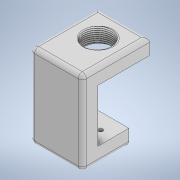
# Autodesk Inventor part: Clamp_Main_Body
Saved by Autodesk Inventor 2021 (Build 250183000, 183)
## iProperties
Created: 2021-04-05
Part Number: Clamp_Main_Body
Material: Generic
Document SubType Name: Modeling
Designer: Ariel Wolle
Density: 1 g/cm^3
Appearance: Default
Author: Ariel Wolle
Autodesk Inventor part; units mm, degrees
ref_plane "YZ Plane" through (0, 0, 0) normal (1, 0, 0) x (0, 1, 0)
ref_plane "XZ Plane" through (0, 0, 0) normal (0, 1, 0) x (-1, 0, 0)
ref_plane "XY Plane" through (0, 0, 0) normal (0, 0, 1) x (1, 0, 0)
sketch "Sketch1" plane through (0, 0, 0) normal (0, 0, 1) x (1, 0, 0)
  line L0 (130, -15) -> (80, -15)
  line L1 (80, -15) -> (80, 27.7)
  line L2 (80, 27.7) -> (130, 27.7)
  line L3 (130, 27.7) -> (130, -15)
  point P0 (0, 0)
  dimension "d0" = 42.7
  dimension "d1" = 15
  dimension "d2" = 80
  dimension "d3" = 50
  constraints: 8 end point, 2 parallel, 1 horizontal, 1 perpendicular
  measures "d0" distance of L2.end L0.start
  measures "d1" distance from line of point (0, 0) L0
  measures "d2" distance from line of point (0, 0) L1
  measures "d3" distance of L0.start L0.end
extrude "Extrusion1" add sketch "Sketch1" along normal blind 15
sketch "Sketch2" plane through (0, 0, 0) normal (0, 0, -1) x (-1, 0, 0)
  line L0 (-80, -15) -> (-130, -15) projected
  line L1 (-80, 27.7) -> (-80, -15) projected
  line L2 (-130, -15) -> (-80, -15)
  line L3 (-80, -15) -> (-80, 0)
  line L4 (-80, 0) -> (-130, 0)
  line L5 (-130, 0) -> (-130, -15)
  point P0 (0, 0)
  constraints: 8 end point, 2 parallel, 1 horizontal, 1 perpendicular, 1 point on line
extrude "Extrusion2" add sketch "Sketch2" along normal blind 30
sketch "Sketch3" plane through (80, -15, 15) normal (0, -1, 0) x (1, 0, 0)
  circle A0 centre (12, -29.7778) radius 2
  circle A1 centre (38, -29.7778) radius 2.1598
  line L0 (0, -45) -> (0, 0) projected
  line L1 (50, -45) -> (50, 0) projected
  point P0 (-80, -15)
  dimension "d8" = 4
  dimension "d9" = 12
  dimension "d10" = 12
  constraints: 2 centre point
  measures "d8" diameter of A0
  measures "d9" distance from line of L0 A0.centre
  measures "d10" distance from line of L1 A1.centre
extrude "Extrusion3" cut sketch "Sketch3" against normal blind 30
chamfer "Chamfer1" distance 2 angle 45 2 edges at (90, -15, -14.7778) (115.8402, -15, -14.7778)
fillet "Fillet1" radius 4 1 edges at (105, -15, 15)
sketch "Sketch4" plane through (80, 27.7, 0) normal (0, 1, 0) x (1, 0, 0)
  line L0 (50, -11) -> (50, -15) projected
  line L1 (0, 0) -> (0, 30) projected
  line L2 (50, -15) -> (0, -15)
  line L3 (0, -15) -> (0, 0)
  line L4 (0, 0) -> (50, 0)
  line L5 (50, 0) -> (50, -15)
  point P0 (-80, 0)
  constraints: 8 end point, 2 parallel, 1 horizontal, 1 perpendicular
extrude "Extrusion4" add sketch "Sketch4" along normal blind 23.1
sketch "Sketch5" plane through (80, 50.8, 0) normal (0, 1, 0) x (1, 0, 0)
  line L0 (0, -15) -> (0, -11) projected
  line L1 (50, 0) -> (50, 30) projected
  line L2 (0, -15) -> (50, -15)
  line L3 (50, -15) -> (50, 0)
  line L4 (50, 0) -> (0, 0)
  line L5 (0, 0) -> (0, -15)
  point P0 (-80, 0)
  point P1 (0, -11)
  constraints: 8 end point, 2 parallel, 1 horizontal, 1 perpendicular
extrude "Extrusion5" add sketch "Sketch5" along normal blind 15
sketch "Sketch6" plane through (0, 0, 0) normal (0, 0, -1) x (-1, 0, 0)
  line L0 (-130, 65.8) -> (-80, 65.8) projected
  line L1 (-130, 0) -> (-130, 65.8) projected
  line L2 (-80, 65.8) -> (-130, 65.8)
  line L3 (-130, 65.8) -> (-130, 50.8)
  line L4 (-130, 50.8) -> (-80, 50.8)
  line L5 (-80, 50.8) -> (-80, 65.8)
  point P0 (0, 0)
  dimension "d21" = 15
  constraints: 8 end point, 2 parallel, 1 horizontal, 1 perpendicular, 1 point on line
  measures "d21" distance between parallel lines of L4 L0
extrude "Extrusion6" add sketch "Sketch6" along normal blind 50
sketch "Sketch7" plane through (80, 65.8, 0) normal (0, 1, 0) x (1, 0, 0)
  line L0 (0, 50) -> (50, 50) projected
  line L1 (0, -15) -> (0, 50) projected
  circle A0 centre (25, 25) radius 13.5
  point P0 (-80, 0)
  dimension "d32" = 25
  dimension "d33" = 25
  dimension "d34" = 27
  constraints: 1 centre point, 1 coincident
  measures "d32" distance from line of L0 point (25, 25)
  measures "d33" distance from line of L1 point (25, 25)
  measures "d34" diameter of A0
fillet "Fillet2" radius 4 11 edges at (105, 65.8, 15) (80, 65.8, -17.5) (130, 65.8, -17.5) (105, 65.8, -50) (80, -13.8284, 13.8284) (80, -15, -9.5) (80, 27.4, 15) (130, -13.8284, 13.8284) (130, -15, -9.5) (130, 27.4, 15) (105, -15, -30)
extrude "Extrusion7" cut sketch "Sketch7" against normal up to surface (15 mm away)
ref_plane "Work Plane2" through (0, 0, -25) normal (0, 0, -1) x (-1, 0, 0)
sketch "Sketch8" plane through (0, 0, -25) normal (0, 0, -1) x (-1, 0, 0)
  line L0 (-80, 50.8) -> (-130, 50.8) construction
  line L1 (-89.4629, 50.8) -> (-89.4629, 66.2032) construction
  line L2 (-80, 50.8) -> (-130, 50.8) construction
  line L3 (-130, 0) -> (-130, 50.8) construction
  line L4 (-130, 0) -> (-80, 0) construction
  line L5 (-80, 0) -> (-80, 50.8) construction
  line L6 (-80, 50.8) -> (-80, 61.8) construction
  arc A0 (-126, 65.8) -> (-130, 61.8) centre (-126, 61.8) ccw construction
  line L7 (-126, 65.8) -> (-118.5, 65.8) construction
  line L8 (-118.5, 65.8) -> (-118.5, 50.8) construction
  line L9 (-118.5, 50.8) -> (-130, 50.8) construction
  line L10 (-130, 50.8) -> (-130, 61.8) construction
  arc A1 (-80, 61.8) -> (-84, 65.8) centre (-84, 61.8) ccw construction
  line L11 (-80, 61.8) -> (-80, 50.8) construction
  line L12 (-80, 50.8) -> (-91.5, 50.8) construction
  line L13 (-91.5, 50.8) -> (-91.5, 65.8) construction
  line L14 (-91.5, 65.8) -> (-84, 65.8) construction
  arc A2 (-130, -11) -> (-126, -15) centre (-126, -11) ccw construction
  line L15 (-130, -11) -> (-130, 0) construction
  line L16 (-130, 0) -> (-80, 0) construction
  line L17 (-80, 0) -> (-80, -11) construction
  arc A3 (-84, -15) -> (-80, -11) centre (-84, -11) ccw construction
  line L18 (-84, -15) -> (-126, -15) construction
  arc A4 (-126, 65.8) -> (-130, 61.8) centre (-126, 61.8) ccw construction
  line L19 (-126, 65.8) -> (-118.5, 65.8) construction
  line L20 (-118.5, 50.8) -> (-130, 50.8) construction
  line L21 (-130, 50.8) -> (-130, 61.8) construction
  arc A5 (-80, 61.8) -> (-84, 65.8) centre (-84, 61.8) ccw construction
  line L22 (-80, 61.8) -> (-80, 50.8) construction
  line L23 (-80, 50.8) -> (-91.5, 50.8) construction
  line L24 (-91.5, 65.8) -> (-84, 65.8) construction
  arc A6 (-130, -11) -> (-126, -15) centre (-126, -11) ccw construction
  line L25 (-130, -11) -> (-130, 0) construction
  line L26 (-130, 0) -> (-80, 0) construction
  line L27 (-80, 0) -> (-80, -11) construction
  arc A7 (-84, -15) -> (-80, -11) centre (-84, -11) ccw construction
  line L28 (-84, -15) -> (-126, -15) construction
  arc A8 (-126, 65.8) -> (-130, 61.8) centre (-126, 61.8) ccw construction
  line L29 (-126, 65.8) -> (-118.5, 65.8) construction
  line L30 (-118.5, 50.8) -> (-130, 50.8) construction
  line L31 (-130, 50.8) -> (-130, 61.8) construction
  arc A9 (-80, 61.8) -> (-84, 65.8) centre (-84, 61.8) ccw construction
  line L32 (-80, 61.8) -> (-80, 50.8) construction
  line L33 (-80, 50.8) -> (-91.5, 50.8) construction
  line L34 (-91.5, 65.8) -> (-84, 65.8) construction
  arc A10 (-130, -11) -> (-126, -15) centre (-126, -11) ccw construction
  line L35 (-130, -11) -> (-130, 0) construction
  line L36 (-130, 0) -> (-80, 0) construction
  line L37 (-80, 0) -> (-80, -11) construction
  arc A11 (-84, -15) -> (-80, -11) centre (-84, -11) ccw construction
  line L38 (-84, -15) -> (-126, -15) construction
  line L39 (-91.5, 50.8) -> (-91.5, 48.8) construction
  line L40 (-91.5, 48.8) -> (-91.5, 47.3)
  line L41 (-91.5, 47.3) -> (-89.9994, 47.8627)
  line L42 (-89.9994, 48.2373) -> (-91.5, 48.8)
  line L43 (-91.5, 48.05) -> (-89.5, 48.05) construction
  arc A12 (-89.9994, 47.8627) -> (-89.9994, 48.2373) centre (-90.0696, 48.05) ccw
  line L44 (-118.5, 65.8) -> (-118.5, 50.8) projected
  line L45 (-91.5, 50.8) -> (-91.5, 65.8) projected
  line L46 (-118.5, 65.8) -> (-118.5, 50.8) projected
  line L47 (-91.5, 50.8) -> (-91.5, 65.8) projected
  point P0 (0, 0)
  dimension "d38" = 2
  dimension "d39" = 0.75
  dimension "d40" = 2
  dimension "d41" = 0.2
  constraints: 12 end point, 3 point on line, 3 vertical, 2 point on circle, 2 tangent, 1 centre point, 1 midpoint, 1 perpendicular
  measures "d38" distance from line of L0 L39.end
  measures "d39" distance from line of L43 L39.end
  measures "d40" distance from line of L40 L43.end
  measures "d41" radius of A12
coil "Coil1" sketch "Sketch8" operation cut axis through (105, 65.8, -25) along (0, 1, 0) pitch 1.7 turns 33.382353 hand right
body "Solid1"
